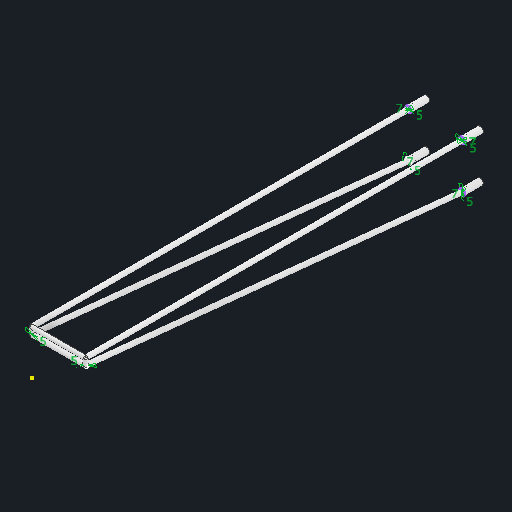
# Autodesk Inventor part: RCPlaneSkeletonTail1
Saved by Autodesk Inventor 2026.1 (Build 301233000, 233)
## iProperties
Created: 2026-02-24
Part Number: RCPlaneSkeletonTail1
Material: PC/ABS Plastic
Document SubType Name: Modeling
Designer: morri
Density: 1.1 g/cm^3
Appearance: Smooth - White
Mass: 40.3226 g
Surface Area: 312.404 cm^2
Volume: 36.6569 cm^3
Author: morri
Autodesk Inventor part; units mm, degrees
sketch "FRONT" plane through (0, 0, 0) normal (0, 0, 1) x (1, 0, 0)
  circle A0 centre (0, 0) radius 3.5
  circle A1 centre (0, 50) radius 3.5
  circle A2 centre (60, 50) radius 3.5
  circle A3 centre (60, 0) radius 3.5
  circle A4 centre (0, 50) radius 2.5
  circle A5 centre (60, 50) radius 2.5
  circle A6 centre (0, 0) radius 2.5
  circle A7 centre (60, 0) radius 2.5
  dimension "d0" = 7
  dimension "d3" = 7
  dimension "d4" = 7
  dimension "d5" = 7
  dimension "d23" = 5
  dimension "d24" = 5
  dimension "d25" = 5
  dimension "d26" = 5
  constraints: 8 centre point, 5 coincident
  measures "d0" diameter of A0
  measures "d3" diameter of A1
  measures "d4" diameter of A3
  measures "d5" diameter of A2
  measures "d23" diameter of A4
  measures "d24" diameter of A5
  measures "d25" diameter of A6
  measures "d26" diameter of A7
extrude "Connectors" add sketch "FRONT" against normal blind 20.3 contours A0 | A1 | A2 | A3 | A4 | A5 | A6 | A7
ref_plane "Work Plane1" through (0, 0, -20.3) normal (0, 0, -1) x (-1, 0, 0)
sketch "Sketch2" plane through (0, 0, -20.3) normal (0, 0, -1) x (-1, 0, 0)
  circle A0 centre (0, 0) radius 3.5 projected
  circle A1 centre (0, 50) radius 3.5 projected
  circle A2 centre (-60, 50) radius 3.5 projected
  circle A3 centre (-60, 0) radius 3.5 projected
  constraints: 4 coincident
hole "Hole1" at (60, 0, -20.3) at (60, 50, -20.3) at (0, 50, -20.3) at (0, 0, -20.3) direction (0, 0, 1) diameter 5.3 depth 15.3
extrude "LongTop" add sketch "FRONT" along normal blind 420 contours A4 | A5
sketch "Sketch5" plane through (0, 0, 0) normal (1, 0, 0) x (0, 1, 0)
  line L0 (52.5, 420) -> (47.5, 420) projected
  circle A0 centre (50, 420) radius 2.5
  circle A1 centre (42.5, 420) radius 2.5
  point P0 (0, 0)
  dimension "d29" = 5
  dimension "d31" = 5
  constraints: 2 centre point, 1 midpoint
  measures "d29" diameter of A0
  measures "d31" diameter of A1
extrude "BackSide" add sketch "Sketch5" along normal blind 60 contours L0 A0 | A1 picked at (49.8996, 420.8273)
ref_plane "Work Plane2" through (0, 50, 422.5) normal (0, 1, 0) x (-1, 0, 0)
sketch "Sketch6" plane through (0, 50, 422.5) normal (0, 1, 0) x (-1, 0, 0)
  line L0 (2.5, -2.5) -> (0, -2.5) projected
  line L1 (0, 0) -> (0, -2.5) projected
  circle A0 centre (0, -2.5) radius 2.5
  line L2 (-60, -2.5) -> (-62.5, -2.5) projected
  circle A1 centre (-60, -2.5) radius 2.5
  point P0 (0, -422.5)
  dimension "d34" = 5
  dimension "d35" = 5
  constraints: 1 centre point, 1 vertical alignment, 2 other
  measures "d35" diameter of A1
extrude "BackDown" add sketch "Sketch6" against normal blind 7.5
ref_plane "TAILXY" through (62.5, 50, 420) normal (0, 0, 1) x (1, 0, 0)
sketch "Sketch7" plane through (62.5, 50, 420) normal (0, 0, 1) x (1, 0, 0)
  line L0 (-65, -7.5) -> (-62.5, -7.5) projected
  circle A0 centre (-62.5, -7.5) radius 2.5
  line L1 (-2.5, -7.5) -> (0, -7.5) projected
  circle A1 centre (-2.5, -7.5) radius 2.5
  point P0 (-62.5, -50)
  dimension "d38" = 5
  dimension "d39" = 5
  constraints: 2 centre point
  measures "d38" diameter of A0
  measures "d39" diameter of A1
sketch3d "3D Sketch1"
  line L0 (60, 0, 0) -> (60, 42.5, 420)
sweep "Sweep1" add profiles "FRONT" path "3D Sketch1" contours A6 | A7
equation "\"Fit_Tolerance\" = 0.3"
